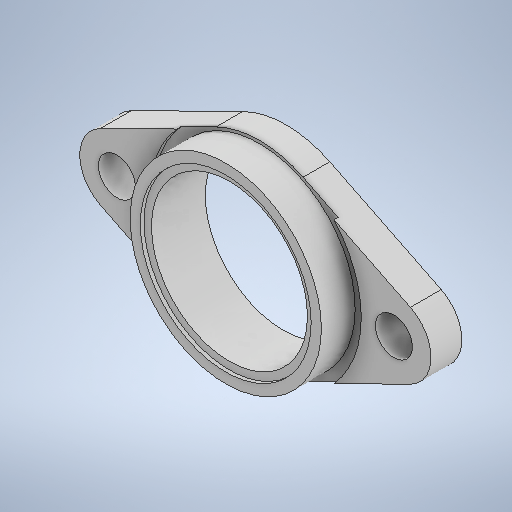
# Autodesk Inventor part: Flange
Saved by Autodesk Inventor 2025.2 (Build 292293000, 293)
## iProperties
Created: 2021-04-20
Part Number: Flange
Material: Generic
Document SubType Name: Modeling
Designer: Johnson Ebenezer R
Density: 1 g/cm^3
Appearance: Default
Author: Johnson Ebenezer R
Autodesk Inventor part; units mm, degrees
ref_plane "YZ Plane" through (0, 0, 0) normal (1, 0, 0) x (0, 1, 0)
ref_plane "XZ Plane" through (0, 0, 0) normal (0, 1, 0) x (-1, 0, 0)
ref_plane "XY Plane" through (0, 0, 0) normal (0, 0, 1) x (1, 0, 0)
sketch "Sketch1" plane through (0, 0, 0) normal (0, 0, 1) x (1, 0, 0)
  line L0 (-18.65, 0) -> (18.65, 0) construction
  line L1 (-18.65, -5) -> (18.65, -5) construction
  line L2 (18.65, 5) -> (-18.65, 5) construction
  arc A0 (-18.65, 5) -> (-18.65, -5) centre (-18.65, 0) ccw
  arc A1 (18.65, -5) -> (18.65, 5) centre (18.65, 0) ccw
  circle A2 centre (0, 0) radius 13.25
  circle A3 centre (-18.65, 0) radius 2.5
  circle A4 centre (18.65, 0) radius 2.5
  line L3 (-20.8618, 4.4842) -> (-5.8613, 11.8831)
  line L4 (20.8618, 4.4842) -> (5.8613, 11.8831)
  line L5 (-20.8618, -4.4842) -> (-5.8613, -11.8831)
  line L6 (5.8613, -11.8831) -> (20.8618, -4.4842)
  circle A5 centre (0, 0) radius 10.5
  dimension "d0" = 47.3
  dimension "d1" = 26.5
  dimension "d2" = 5
  dimension "d3" = 2.5
  dimension "d4" = 21
  constraints: 16 end point, 12 point on circle, 12 tangent, 6 centre point, 4 coincident, 1 equal radius, 1 horizontal, 1 midpoint, 1 parallel
  measures "d1" diameter of A2
  measures "d2" diameter of A3
  measures "d3" radial gap between concentric circles of A0 A3
  measures "d4" diameter of A5
extrude "Extrusion1" add sketch "Sketch1" along normal blind 4.15
sketch "Sketch2" plane through (0, 0, 4.15) normal (0, 0, 1) x (1, 0, 0)
  circle A0 centre (0, 0) radius 14.25
  dimension "d7" = 28.5
  constraints: 1 centre point, 1 coincident
  measures "d7" diameter of A0
extrude "Extrusion2" cut sketch "Sketch2" against normal blind 0.55
sketch "Sketch3" plane through (0, 0, 0) normal (0, 0, -1) x (-1, 0, 0)
  arc A0 (-5.8613, -11.8831) -> (5.8613, -11.8831) centre (0, 0) ccw projected
  line L0 (20.8618, -4.4842) -> (5.8613, -11.8831) projected
  arc A1 (20.8618, -4.4842) -> (20.8618, 4.4842) centre (18.65, 0) ccw projected
  line L1 (5.8613, 11.8831) -> (20.8618, 4.4842) projected
  arc A2 (5.8613, 11.8831) -> (-5.8613, 11.8831) centre (0, 0) ccw projected
  line L2 (-20.8618, 4.4842) -> (-5.8613, 11.8831) projected
  arc A3 (-20.8618, 4.4842) -> (-20.8618, -4.4842) centre (-18.65, 0) ccw projected
  line L3 (-5.8613, -11.8831) -> (-20.8618, -4.4842) projected
  circle A4 centre (0, 0) radius 10.5 projected
  circle A5 centre (-18.65, 0) radius 2.5 projected
  circle A6 centre (18.65, 0) radius 2.5 projected
  arc A7 (5.1977, 10.5378) -> (-5.1977, 10.5378) centre (0, 0) ccw
  line L4 (5.1977, 10.5378) -> (20.1983, 3.1389)
  arc A8 (20.1983, -3.1389) -> (20.1983, 3.1389) centre (18.65, 0) ccw
  line L5 (20.1983, -3.1389) -> (5.1977, -10.5378)
  arc A9 (-5.1977, -10.5378) -> (5.1977, -10.5378) centre (0, 0) ccw
  line L6 (-5.1977, -10.5378) -> (-20.1983, -3.1389)
  arc A10 (-20.1983, 3.1389) -> (-20.1983, -3.1389) centre (-18.65, 0) ccw
  line L7 (-20.1983, 3.1389) -> (-5.1977, 10.5378)
  circle A11 centre (-18.65, 0) radius 4.5
  circle A12 centre (18.65, 0) radius 4.5
  circle A13 centre (-14.4614, 4.296) radius 1.5
  circle A14 centre (14.4614, 4.296) radius 1.5
  circle A15 centre (-14.4614, -4.296) radius 1.5
  circle A16 centre (14.4614, -4.296) radius 1.5
  arc A17 (-16.1071, 5.1569) -> (-16.1905, 3.7684) centre (-15.753, 4.4389) ccw
  line L8 (0, -13.25) -> (0, 13.25) construction
  arc A18 (16.1905, 3.7684) -> (16.1071, 5.1569) centre (15.753, 4.4389) ccw
  arc A19 (-20.8618, 4.4842) -> (-20.8618, -4.4842) centre (-18.65, 0) ccw projected
  arc A20 (20.8618, -4.4842) -> (20.8618, 4.4842) centre (18.65, 0) ccw projected
  line L9 (-23.65, 0) -> (23.65, 0) construction
  arc A21 (-16.1905, -3.7684) -> (-16.1071, -5.1569) centre (-15.753, -4.4389) ccw
  arc A22 (16.1071, -5.1569) -> (16.1905, -3.7684) centre (15.753, -4.4389) ccw
  point P0 (-15.125, 5.6413)
  point P1 (-15.5086, 3.222)
  point P2 (-15.5086, -3.222)
  point P3 (-15.125, -5.6413)
  point P4 (15.125, -5.6413)
  point P5 (15.5086, -3.222)
  point P6 (15.5086, 3.222)
  point P7 (15.125, 5.6413)
  point P8 (16.1071, -5.1569)
  point P9 (16.1905, -3.7684)
  point P10 (-16.1905, -3.7684)
  point P11 (-16.1071, -5.1569)
  point P12 (16.1905, 3.7684)
  point P13 (16.1071, 5.1569)
  dimension "d10" = 1.5
  dimension "d11" = 2
  dimension "d13" = 3
  dimension "d15" = 0.6
  constraints: 20 point on circle, 13 centre point, 12 end point, 9 symmetric about line, 4 tangent, 3 equal radius, 2 horizontal alignment, 2 vertical alignment, 1 point on line, 16 other
  measures "d10" distance between parallel lines of L7 L2
  measures "d13" diameter of A13
extrude "Extrusion3" cut sketch "Sketch3" against normal blind 0.4 contours L4 A14 A12 A16 L5 A9 L6 A15 A11 A13 L7 A7 | L4 A18 A12 A14 | A13 A11 A17 L7 | A12 A22 L5 A16 | A15 L6 A21 A11
sketch "Sketch4" plane through (0, 0, 0.4) normal (0, 0, -1) x (-1, 0, 0)
  line L0 (-13.4137, 6.2066) -> (-11.7284, 7.0379) construction
  line L1 (-11.7284, 7.0379) -> (-11.0649, 5.6926) construction
  line L2 (-11.0649, 5.6926) -> (-12.7502, 4.8614) construction
  line L3 (-12.7502, 4.8614) -> (-13.4137, 6.2066) construction
  line L4 (-15.125, 5.6413) -> (-5.1977, 10.5378) construction
  line L5 (-15.125, 5.6413) -> (-5.1977, 10.5378) construction
  arc A0 (-15.5086, 3.222) -> (-15.125, 5.6413) centre (-14.4614, 4.296) ccw construction
  arc A1 (-15.5086, -3.222) -> (-15.5086, 3.222) centre (-18.65, 0) ccw construction
  arc A2 (-15.125, -5.6413) -> (-15.5086, -3.222) centre (-14.4614, -4.296) ccw construction
  line L6 (-5.1977, -10.5378) -> (-15.125, -5.6413) construction
  arc A3 (-5.1977, -10.5378) -> (5.1977, -10.5378) centre (0, 0) ccw construction
  line L7 (15.125, -5.6413) -> (5.1977, -10.5378) construction
  arc A4 (15.5086, -3.222) -> (15.125, -5.6413) centre (14.4614, -4.296) ccw construction
  arc A5 (15.5086, 3.222) -> (15.5086, -3.222) centre (18.65, 0) ccw construction
  arc A6 (15.125, 5.6413) -> (15.5086, 3.222) centre (14.4614, 4.296) ccw construction
  line L8 (5.1977, 10.5378) -> (15.125, 5.6413) construction
  arc A7 (5.1977, 10.5378) -> (-5.1977, 10.5378) centre (0, 0) ccw construction
  circle A8 centre (0, 0) radius 10.5 construction
  arc A9 (12.4858, 5.828) -> (13.519, 1.9805) centre (14.4614, 4.296) ccw construction
  arc A10 (13.519, 1.9805) -> (15.3623, -4.4092) centre (18.65, 0) ccw construction
  line L9 (15.3623, -4.4092) -> (4.7554, -9.641) construction
  arc A11 (-4.7554, -9.641) -> (4.7554, -9.641) centre (0, 0) ccw construction
  line L10 (-4.7554, -9.641) -> (-12.4858, -5.828) construction
  arc A12 (-12.4858, -5.828) -> (-16.8001, -5.1796) centre (-14.4614, -4.296) ccw construction
  arc A13 (-16.8001, -5.1796) -> (-15.3623, 4.4092) centre (-18.65, 0) ccw construction
  line L11 (-15.3623, 4.4092) -> (-4.7554, 9.641) construction
  arc A14 (4.7554, 9.641) -> (-4.7554, 9.641) centre (0, 0) ccw construction
  line L12 (4.7554, 9.641) -> (12.4858, 5.828) construction
  line L13 (11.2624, 7.2677) -> (13.2202, 6.3021) construction
  line L14 (13.2202, 6.3021) -> (12.5566, 4.9568) construction
  line L15 (12.5566, 4.9568) -> (10.5989, 5.9224) construction
  line L16 (10.5989, 5.9224) -> (11.2624, 7.2677) construction
  line L17 (-12.3944, 6.5115) -> (-13.0201, 6.2028)
  line L18 (-13.0201, 6.2028) -> (-12.833, 5.8235)
  line L19 (-12.833, 5.8235) -> (-12.2334, 6.1192)
  line L20 (-12.2334, 6.1192) -> (-12.1549, 5.96)
  line L21 (-12.1549, 5.96) -> (-12.7545, 5.6643)
  line L22 (-12.7545, 5.6643) -> (-12.4351, 5.0167)
  line L23 (-12.4351, 5.0167) -> (-12.6139, 4.9286)
  line L24 (-12.6139, 4.9286) -> (-13.2774, 6.2738)
  line L25 (-13.2774, 6.2738) -> (-12.4729, 6.6707)
  line L26 (-12.4729, 6.6707) -> (-12.3944, 6.5115)
  line L27 (-10.8696, 5.7889) -> (-11.6491, 5.4044)
  line L28 (-11.6491, 5.4044) -> (-12.3126, 6.7497)
  line L29 (-12.3126, 6.7497) -> (-12.1339, 6.8379)
  line L30 (-12.1339, 6.8379) -> (-11.5488, 5.6518)
  line L31 (-11.5488, 5.6518) -> (-10.9482, 5.9481)
  line L32 (-10.9482, 5.9481) -> (-10.8696, 5.7889)
  spline S0 degree 2 poles (10.987, 6.5236) (11.1003, 6.7533) (11.4025, 7.0169) (11.558, 7.0413) knots 0 0 0 1 2 2 2
  spline S1 degree 2 poles (11.558, 7.0413) (11.679, 7.0622) (11.7746, 7.0151) knots 0 0 0 1 1 1
  spline S2 degree 2 poles (11.7746, 7.0151) (11.9296, 6.9386) (11.9751, 6.7208) knots 0 0 0 1 1 1
  spline S3 degree 2 poles (11.9751, 6.7208) (12.0325, 6.4492) (11.8677, 6.1151) knots 0 0 0 1 1 1
  spline S4 degree 2 poles (11.8677, 6.1151) (11.7523, 5.881) (11.4555, 5.6202) (11.1741, 5.5759) (11.0762, 5.6241) knots 0 0 0 1 2 3 3 3
  spline S5 degree 2 poles (11.0762, 5.6241) (10.8839, 5.719) (10.8675, 6.01) knots 0 0 0 1 1 1
  spline S6 degree 2 poles (10.8675, 6.01) (10.8541, 6.2543) (10.987, 6.5236) knots 0 0 0 1 1 1
  spline S7 degree 2 poles (11.169, 6.4024) (11.0324, 6.1254) (11.0138, 5.9159) knots 0 0 0 1 1 1
  spline S8 degree 2 poles (11.0138, 5.9159) (10.9983, 5.7405) (11.1104, 5.6852) knots 0 0 0 1 1 1
  spline S9 degree 2 poles (11.1104, 5.6852) (11.1643, 5.6586) (11.3258, 5.6978) (11.4113, 5.7964) knots 0 0 0 1 2 2 2
  spline S10 degree 2 poles (11.4113, 5.7964) (11.5415, 5.944) (11.6943, 6.2539) knots 0 0 0 1 1 1
  spline S11 degree 2 poles (11.6943, 6.2539) (11.8082, 6.4847) (11.8363, 6.6608) knots 0 0 0 1 1 1
  spline S12 degree 2 poles (11.8363, 6.6608) (11.8564, 6.793) (11.8236, 6.8679) knots 0 0 0 1 1 1
  spline S13 degree 2 poles (11.8236, 6.8679) (11.7992, 6.921) (11.741, 6.9497) knots 0 0 0 1 1 1
  spline S14 degree 2 poles (11.741, 6.9497) (11.6739, 6.9828) (11.5914, 6.9483) knots 0 0 0 1 1 1
  spline S15 degree 2 poles (11.5914, 6.9483) (11.4793, 6.9011) (11.2536, 6.5738) (11.169, 6.4024) knots 0 0 0 1 2 2 2
  spline S16 degree 2 poles (12.3266, 5.8792) (12.2318, 6.0886) (12.2175, 6.2924) (12.2598, 6.3781) knots 0 0 0 1 2 2 2
  spline S17 degree 2 poles (12.2598, 6.3781) (12.3243, 6.5089) (12.6198, 6.5982) (12.7879, 6.5153) knots 0 0 0 1 2 2 2
  spline S18 degree 2 poles (12.7879, 6.5153) (12.9506, 6.435) (13.0628, 6.1611) (13.007, 6.0479) knots 0 0 0 1 2 2 2
  spline S19 degree 2 poles (13.007, 6.0479) (12.9696, 5.972) (12.7849, 5.8691) (12.563, 5.846) knots 0 0 0 1 2 2 2
  spline S20 degree 2 poles (12.563, 5.846) (12.6716, 5.6257) (12.6892, 5.52) knots 0 0 0 1 1 1
  spline S21 degree 2 poles (12.6892, 5.52) (12.7152, 5.3815) (12.6599, 5.2694) knots 0 0 0 1 1 1
  spline S22 degree 2 poles (12.6599, 5.2694) (12.5899, 5.1276) (12.2742, 5.0333) (12.0984, 5.12) knots 0 0 0 1 2 2 2
  spline S23 degree 2 poles (12.0984, 5.12) (11.906, 5.2149) (11.8585, 5.3872) knots 0 0 0 1 1 1
  spline S24 degree 2 poles (11.8585, 5.3872) (11.8205, 5.5262) (11.8769, 5.6405) knots 0 0 0 1 1 1
  spline S25 degree 2 poles (11.8769, 5.6405) (11.9208, 5.7296) (12.1268, 5.8452) (12.3266, 5.8792) knots 0 0 0 1 2 2 2
  spline S26 degree 2 poles (12.3555, 5.8185) (12.2378, 5.7905) (12.0779, 5.6658) (12.0307, 5.5701) knots 0 0 0 1 2 2 2
  spline S27 degree 2 poles (12.0307, 5.5701) (11.9678, 5.4426) (12.0326, 5.2194) (12.1403, 5.1663) knots 0 0 0 1 2 2 2
  spline S28 degree 2 poles (12.1403, 5.1663) (12.248, 5.1131) (12.4374, 5.1701) (12.4802, 5.2569) knots 0 0 0 1 2 2 2
  spline S29 degree 2 poles (12.4802, 5.2569) (12.5149, 5.3272) (12.5057, 5.4028) knots 0 0 0 1 1 1
  spline S30 degree 2 poles (12.5057, 5.4028) (12.4858, 5.5425) (12.3555, 5.8185) knots 0 0 0 1 1 1
  spline S31 degree 2 poles (12.5353, 5.9088) (12.7077, 5.9563) (12.8327, 6.0491) (12.8712, 6.1271) knots 0 0 0 1 2 2 2
  spline S32 degree 2 poles (12.8712, 6.1271) (12.9227, 6.2315) (12.8631, 6.4072) (12.762, 6.457) knots 0 0 0 1 2 2 2
  spline S33 degree 2 poles (12.762, 6.457) (12.6608, 6.5069) (12.4759, 6.4533) (12.4369, 6.3742) knots 0 0 0 1 2 2 2
  spline S34 degree 2 poles (12.4369, 6.3742) (12.4114, 6.3225) (12.4137, 6.1943) (12.4388, 6.1231) knots 0 0 0 1 2 2 2
  line L33 (12.4388, 6.1231) -> (12.5353, 5.9088)
  point P0 (-13.0819, 5.534)
  point P1 (-11.3967, 6.3652)
  point P2 (12.8884, 5.6294)
  point P3 (10.9307, 6.5951)
  dimension "d18" = 1.5
  dimension "d19" = 1
  dimension "d20" = 1.5
  constraints: 12 point on circle, 8 end point, 6 centre point, 4 midpoint, 4 point on line, 13 other
  measures "d18" distance of L0.end L1.end
  measures "d19" distance between parallel lines of L4 L11
  measures "d20" distance of L13.end L14.end
emboss "Emboss1" sketch "Sketch4" operation add depth 0.4 direction (0, 0, 1)
sketch "Sketch5" plane through (0, 0, 3.6) normal (0, 0, 1) x (1, 0, 0)
  circle A0 centre (0, 0) radius 12.875
  circle A1 centre (0, 0) radius 10.5 projected
  dimension "d24" = 25.75
  constraints: 1 centre point, 1 coincident
  measures "d24" diameter of A0
extrude "Extrusion4" add sketch "Sketch5" along normal blind 4.55
sketch "Sketch6" plane through (0, 0, 8.15) normal (0, 0, 1) x (1, 0, 0)
  circle A0 centre (0, 0) radius 11.5
  dimension "d27" = 23
  constraints: 1 centre point, 1 coincident
  measures "d27" diameter of A0
extrude "Extrusion5" cut sketch "Sketch6" against normal blind 0.5
equation "\"d20\" = d18"
equation "\"d21\" = d16"
equation "\"d16\" = 0.4"
body "Solid1"
